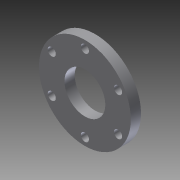
# Autodesk Inventor part: lower box hub
Saved by Autodesk Inventor 2012 (Build 160160000, 160)
## iProperties
Created: 2012-07-17
Part Number: lower box hub
Material: Default
Document SubType Name: Modeling
Designer: Bryce
Density: 1 g/cm^3
Author: Bryce
Autodesk Inventor part; units mm, degrees
ref_plane "YZ Plane" through (0, 0, 0) normal (1, 0, 0) x (0, 1, 0)
ref_plane "XZ Plane" through (0, 0, 0) normal (0, 1, 0) x (-1, 0, 0)
ref_plane "XY Plane" through (0, 0, 0) normal (0, 0, 1) x (1, 0, 0)
sketch "Sketch1" plane through (0, 0, 0) normal (0, 0, 1) x (1, 0, 0)
  circle A0 centre (0, 0) radius 28.575
  circle A1 centre (0, 0) radius 23.8125
  circle A2 centre (0, 0) radius 12.7
  point P0 (20.6222, -11.9063)
  point P1 (20.6222, 11.9062)
  point P2 (0, 23.8125)
  point P3 (-20.6222, 11.9063)
  point P4 (-20.6222, -11.9062)
  point P5 (0, -23.8125)
  dimension "d1" = 47.625
  dimension "d0" = 57.15
  dimension "d4" = 360
  dimension "d6" = 25.4
  constraints: 3 coincident, 2 centre point, 1 vertical alignment, 10 other
  measures "d0" diameter of A0
  measures "d6" diameter of A2
extrude "Extrusion1" add sketch "Sketch1" along normal blind 6.35 contours A0 | A1
hole "Hole1" at (20.6222, -11.9063, 0) at (20.6222, 11.9062, 0) at (0, 23.8125, 0) at (-20.6222, 11.9063, 0) at (-20.6222, -11.9062, 0) at (0, -23.8125, 0) direction (0, 0, 1) diameter 5.08 end through all
body "Solid1"
